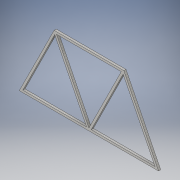
# Autodesk Inventor part: Truss 3Tri
Saved by Autodesk Inventor 2016 (Build 200138000, 138)
## iProperties
Created: 2016-01-30
Part Number: Truss 3Tri
Material: Generic
Document SubType Name: Modeling
Designer: Kurtis
Density: 1 g/cm^3
Appearance: Default
Author: Kurtis
Autodesk Inventor part; units mm, degrees
ref_plane "YZ Plane" through (0, 0, 0) normal (1, 0, 0) x (0, 1, 0)
ref_plane "XZ Plane" through (0, 0, 0) normal (0, 1, 0) x (-1, 0, 0)
ref_plane "XY Plane" through (0, 0, 0) normal (0, 0, 1) x (1, 0, 0)
sketch "Sketch1" plane through (0, 0, 0) normal (0, 0, 1) x (1, 0, 0)
  line L0 (0, 0) -> (203.2, 0)
  line L1 (152.5934, 101.6) -> (50.8, 101.6)
  line L2 (101.6, 0) -> (76.2, 0) construction
  line L3 (127, 101.6) -> (152.5934, 101.6)
  line L4 (0, 0) -> (3.175, 0) construction
  line L5 (152.5934, 101.6) -> (203.2, 0)
  line L6 (50.8, 101.6) -> (0, 0)
  line L7 (52.5749, 98.425) -> (52.6684, 98.2373)
  line L8 (31.4673, 0) -> (31.4673, 3.175) construction
  line L9 (31.4673, 3.175) -> (5.1373, 3.175)
  line L10 (22.7402, 38.3809) -> (5.1373, 3.175)
  line L11 (5.1373, 3.175) -> (51.6882, 96.6446)
  line L12 (176.1115, 47.2628) -> (198.0715, 3.175)
  line L13 (176.1115, 47.2628) -> (151.5146, 96.6447)
  line L14 (54.3484, 98.425) -> (148.8543, 98.425)
  line L15 (66.9801, 65.9439) -> (98.245, 3.175) construction
  line L16 (98.245, 3.175) -> (51.6882, 96.6446)
  line L17 (69.822, 67.3595) -> (54.3484, 98.425)
  line L18 (69.822, 67.3595) -> (101.6, 3.5605)
  line L19 (129.9466, 60.4672) -> (148.8543, 98.425)
  line L20 (132.7885, 59.0516) -> (151.5146, 96.6447)
  line L21 (148.8543, 98.425) -> (101.6, 3.5605)
  line L22 (132.7885, 59.0516) -> (104.9551, 3.175)
  line L23 (98.245, 3.175) -> (31.4673, 3.175)
  line L24 (201.6185, 3.175) -> (104.9551, 3.175)
  dimension "d0" = 203.2
  dimension "d40" = 3.175
  dimension "d42" = 3.175
  dimension "d44" = 3.175
  dimension "d45" = 3.175
  dimension "d51" = 101.6
  dimension "d52" = 93.4696
  dimension "d53" = 94.5059
  dimension "d54" = 96.6634
  constraints: 50 end point, 9 parallel, 9 point on line, 1 horizontal, 1 midpoint, 1 perpendicular, 1 vertical
  measures "d0" distance of L0.start L0.end
  measures "d40" distance of L8.start L8.end
  measures "d42" distance between parallel lines of L6 L10
  measures "d44" distance between parallel lines of L1 L14
  measures "d45" distance between parallel lines of L13 L5
  measures "d51" vertical distance of L1.end L0.start
  measures "d52" vertical distance of L9.end L11.end
  measures "d53" distance of L14.end L14.start
  measures "d54" distance of L24.start L22.end
extrude "Extrusion2" add sketch "Sketch1" along normal blind 3.175
body "Solid2"
